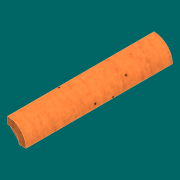
# Autodesk Inventor part: sideMoulding
Saved by Autodesk Inventor 2016 SP1 (Build 200210100, 210)
## iProperties
Created: 2016-04-01
Part Number: sideMoulding
Material: Wood (Cherry)
Document SubType Name: Modeling
Designer: sawai
Density: 0.63 g/cm^3
Appearance: Cherry - Natural Low Gloss
Author: sawai
Autodesk Inventor part; units mm, degrees
ref_plane "YZ Plane" through (0, 0, 0) normal (1, 0, 0) x (0, 1, 0)
ref_plane "XZ Plane" through (0, 0, 0) normal (0, 1, 0) x (-1, 0, 0)
ref_plane "XY Plane" through (0, 0, 0) normal (0, 0, 1) x (1, 0, 0)
sketch "Sketch1" plane through (0, 0, 0) normal (1, 0, 0) x (0, 1, 0)
  line L0 (-6.35, 6.35) -> (6.35, 6.35)
  line L1 (6.35, 6.35) -> (6.35, -6.35)
  line L2 (6.35, -6.35) -> (-6.35, -6.35)
  line L3 (-6.35, -6.35) -> (-6.35, 6.35)
  line L4 (-6.35, 6.35) -> (6.35, -6.35) construction
  line L5 (6.35, 6.35) -> (-6.35, -6.35) construction
  point P0 (0, 0)
  dimension "d0" = 12.7
  dimension "d1" = 12.7
  constraints: 12 end point, 2 midpoint, 2 parallel, 1 horizontal, 1 perpendicular
  measures "d0" distance of L1.end L2.end
  measures "d1" distance of L0.end L1.end
extrude "Extrusion1" add sketch "Sketch1" along normal mid plane 100
chamfer "Chamfer1" distance 6.35 angle 45 1 edges at (0, -6.35, -6.35)
fillet "Fillet1" radius 12.7 1 edges at (0, 6.35, 6.35)
sketch "Sketch2" plane through (50, 0, -6.35) normal (0, 0, -1) x (-1, 0, 0)
  line L0 (100, 0) -> (0, 0) projected
  line L1 (100, 6.35) -> (100, 0) projected
  line L2 (0, 6.35) -> (100, 6.35) projected
  line L3 (0, 0) -> (0, 6.35) projected
  circle A0 centre (100, 0) radius 1.5875
  line L4 (0, -6.35) -> (100, -6.35) projected
  line L5 (100, 0) -> (0, 0) projected
  line L6 (98.4125, 0) -> (98.4125, -6.35)
  line L7 (101.5875, 0) -> (101.5875, -6.35)
  line L8 (101.5875, -6.35) -> (98.4125, -6.35)
  point P0 (50, 0)
  dimension "d8" = 3.175
  constraints: 6 end point, 2 perpendicular, 2 point on circle, 2 point on line, 2 tangent, 1 centre point, 1 coincident, 1 vertical
  measures "d8" diameter of A0
revolve "Revolution1" cut sketch "Sketch2" angle 360 about axis through (50, -6.35, -6.35) along (-1, 0, 0) contours L1 A0 L0 | L0 A0 L1 | A0 L7 L8 L4 L6
mirror "Mirror1" about plane through (0, 0, 0) normal (1, 0, 0) of "Revolution1"
equation "\"d0\" = facingThickness"
equation "\"d1\" = facingThickness"
equation "\"d2\" = depth"
equation "\"d4\" = 0.5 * facingThickness"
equation "\"d7\" = facingThickness"
equation "\"d8\" = 0.25 * facingThickness"
equation "\"mppcMountThickness\" = 6.35"
equation "\"depth\" = 100"
equation "\"facingThickness\" = 12.7"
equation "\"facingGasketThickness\" = 1.5875"
body "Solid1"
